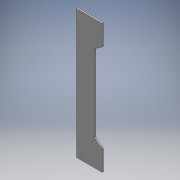
# Autodesk Inventor part: Coté long plateau - 2
Saved by Autodesk Inventor 2016 SP1 (Build 200210100, 210)
## iProperties
Created: 2017-04-25
Part Number: Coté long plateau - 2
Material: Bois (bouleau)
Document SubType Name: Modeling
Designer: dimercur
Density: 0.55 g/cm^3
Appearance: Par défaut
Author: dimercur
Autodesk Inventor part; units mm, degrees
ref_plane "YZ Plane" through (0, 0, 0) normal (1, 0, 0) x (0, 1, 0)
ref_plane "XZ Plane" through (0, 0, 0) normal (0, 1, 0) x (-1, 0, 0)
ref_plane "XY Plane" through (0, 0, 0) normal (0, 0, 1) x (1, 0, 0)
sketch "Esquisse1" plane through (0, 0, 0) normal (0, 1, 0) x (-1, 0, 0)
  line L0 (100, 500) -> (-100, 500)
  line L1 (-100, 500) -> (-100, -500)
  line L2 (-100, -500) -> (100, -500)
  line L3 (100, -500) -> (100, 500)
  point P0 (0, 0)
  dimension "d0" = 1000
  dimension "d1" = 200
  dimension "d4" = 500
  dimension "d5" = 100
  constraints: 8 end point, 2 parallel, 1 horizontal, 1 perpendicular
  measures "d0" distance of L2.end L0.start
  measures "d1" distance of L0.start L0.end
  measures "d4" vertical distance of point (0, 0) L0.start
  measures "d5" horizontal distance of point (0, 0) L0.start
extrude "Extrusion1" add sketch "Esquisse1" along normal blind 10
sketch "Esquisse2" plane through (0, 10, 0) normal (0, 1, 0) x (1, 0, 0)
  line L0 (100, -500) -> (100, 500) projected
  line L1 (100, -340) -> (40, -300)
  line L2 (40, -300) -> (40, 300)
  line L3 (40, 300) -> (100, 340)
  line L4 (-100, 500) -> (-100, -500) projected
  point P0 (0, 0)
  dimension "d6" = 600
  dimension "d7" = 300
  dimension "d8" = 140
  dimension "d9" = 160
  dimension "d10" = 160
  constraints: 6 end point, 2 point on line, 1 parallel
  measures "d6" distance of L1.end L2.end
  measures "d7" vertical distance of point (0, 0) L1.end
  measures "d8" distance from line of L4 L1.end
  measures "d9" distance of L0.start L1.start
  measures "d10" distance of L0.end L3.end
extrude "Extrusion2" cut sketch "Esquisse2" against normal through all
fillet "Congé1" radius 20 4 edges at (40, 5, 300) (100, 5, 340) (40, 5, -300) (100, 5, -340)
sketch "Esquisse3" plane through (0, 10, 0) normal (0, 1, 0) x (1, 0, 0)
  circle A0 centre (-60, -485) radius 1.5
  circle A1 centre (60, -485) radius 1.5
  circle A2 centre (-60, 485) radius 1.5
  circle A3 centre (60, 485) radius 1.5
  line L0 (-100, -500) -> (100, -500) projected
  line L1 (100, 500) -> (-100, 500) projected
  line L2 (-100, 500) -> (-100, -500) projected
  line L3 (100, -500) -> (100, -350.7037) projected
  line L4 (100, 350.7037) -> (100, 500) projected
  point P0 (0, 0)
  dimension "d14" = 3
  dimension "d15" = 3
  dimension "d16" = 3
  dimension "d17" = 3
  dimension "d18" = 15
  dimension "d19" = 15
  dimension "d20" = 15
  dimension "d21" = 15
  dimension "d22" = 40
  dimension "d23" = 40
  dimension "d24" = 40
  dimension "d25" = 40
  constraints: 4 centre point
  measures "d14" diameter of A0
  measures "d15" diameter of A1
  measures "d16" diameter of A3
  measures "d17" diameter of A2
  measures "d18" distance from line of L0 A0.centre
  measures "d19" distance from line of L1 A2.centre
  measures "d20" distance from line of L1 A3.centre
  measures "d21" distance from line of L0 A1.centre
  measures "d22" distance from line of L2 A0.centre
  measures "d23" distance from line of L3 A1.centre
  measures "d24" distance from line of L2 A2.centre
  measures "d25" distance from line of L4 A3.centre
extrude "Extrusion3" cut sketch "Esquisse3" against normal through all
equation "\"d4\" = 0.5 * d0"
equation "\"d5\" = 0.5 * d1"
equation "\"d7\" = 0.5 * d6"
equation "\"d10\" = d9"
equation "\"d15\" = d14"
equation "\"d16\" = d14"
equation "\"d17\" = d14"
equation "\"d19\" = d18"
equation "\"d20\" = d18"
equation "\"d21\" = d18"
equation "\"d23\" = d22"
equation "\"d24\" = d22"
equation "\"d25\" = d22"
